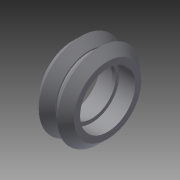
# Autodesk Inventor part: Rail_OpenVWheel
Saved by Autodesk Inventor 2014 (Build 180170000, 170)
## iProperties
Created: 2014-01-09
Part Number: Rail_OpenVWheel
Material: Acetal Resin, Black
Document SubType Name: Modeling
Designer: ThatOtherGuy
Density: 1.425 g/cm^3
Mass: 2.60637 g
Surface Area: 18.3029 cm^2
Volume: 1.82903 cm^3
Appearance: Smooth - Black
Author: ThatOtherGuy
Autodesk Inventor part; units mm, degrees
ref_plane "YZ Plane" through (0, 0, 0) normal (1, 0, 0) x (0, 1, 0)
ref_plane "XZ Plane" through (0, 0, 0) normal (0, 1, 0) x (-1, 0, 0)
ref_plane "XY Plane" through (0, 0, 0) normal (0, 0, 1) x (1, 0, 0)
sketch "Sketch1" plane through (0, 0, 0) normal (0, 0, 1) x (1, 0, 0)
  line L0 (-2.42, 21.97) -> (-2.42, 2.42)
  line L1 (-2.42, 2.42) -> (0, 0)
  line L2 (0, 0) -> (2.42, 2.42)
  line L3 (2.42, 2.42) -> (2.42, 2.82)
  line L4 (2.42, 2.82) -> (2.97, 2.82)
  line L5 (2.97, 2.82) -> (2.97, 2.42)
  line L6 (2.97, 2.42) -> (5.39, 0)
  line L7 (5.39, 0) -> (7.81, 2.42)
  line L8 (7.81, 2.42) -> (7.81, 21.97)
  line L9 (7.81, 21.97) -> (5.39, 24.39)
  line L10 (5.39, 24.39) -> (2.97, 21.97)
  line L11 (2.97, 21.97) -> (2.97, 21.57)
  line L12 (2.97, 21.57) -> (2.42, 21.57)
  line L13 (2.42, 21.57) -> (2.42, 21.97)
  line L14 (2.42, 21.97) -> (0, 24.39)
  line L15 (0, 24.39) -> (-2.42, 21.97)
  line L16 (7.81, 12.195) -> (-2.42, 12.195)
  line L17 (-2.42, 20.195) -> (2.195, 20.195)
  line L18 (2.195, 20.195) -> (2.195, 19.14)
  line L19 (2.195, 19.14) -> (3.195, 19.14)
  line L20 (3.195, 19.14) -> (3.195, 20.195)
  line L21 (3.195, 20.195) -> (7.81, 20.195)
  line L22 (-2.42, 4.195) -> (2.195, 4.195)
  line L23 (3.195, 4.195) -> (7.81, 4.195)
  line L24 (3.195, 4.195) -> (3.195, 5.25)
  line L25 (3.195, 5.25) -> (2.195, 5.25)
  line L26 (2.195, 5.25) -> (2.195, 4.195)
  dimension "d0" = 24.39
  dimension "d2" = 10.23
  dimension "d3" = 5.39
  dimension "d4" = 18.75
  dimension "d7" = 90
  dimension "d8" = 12.195
  dimension "d15" = 1
  dimension "d17" = 13.89
  dimension "d18" = 16
  dimension "d19" = 8
  constraints: 54 end point, 15 equal length, 11 parallel, 8 horizontal alignment, 6 perpendicular, 4 point on line, 2 midpoint, 1 coincident, 1 horizontal, 1 vertical
  measures "d0" distance of L6.end L9.end
  measures "d2" distance between parallel lines of L8 L0
  measures "d3" distance of L9.end L14.end
  measures "d4" distance between parallel lines of L4 L12
  measures "d7" angle of L2 L1
  measures "d8" vertical distance of L6.end L16.start
  measures "d15" distance of L18.end L19.end
  measures "d17" distance between parallel lines of L19 L25
  measures "d18" distance between parallel lines of L23 L21
  measures "d19" distance between parallel lines of L16 L21
revolve "Revolution1" add sketch "Sketch1" angle 360 about axis through (7.81, 12.195, 0) along (-1, 0, 0) contours L22 L26 L25 L24 L23 L8 L7 L6 L5 L4 L3 L2 L1 L0
equation "\"d8\" = 0.5 * d0"
equation "\"d19\" = 0.5 * d18"
body "Solid1"
